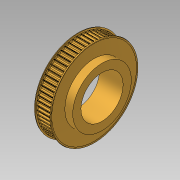
# Autodesk Inventor part: Engine Belt Wheel-2
Saved by Autodesk Inventor 2018.2 (Build 222227000, 227)
## iProperties
Created: 2019-08-01
Part Number: Engine Belt Wheel-2
Material: Generic
Document SubType Name: Modeling
Designer: NiveshandNisheeth
Density: 1 g/cm^3
Appearance: Brass - Satin
Author: NiveshandNisheeth
Autodesk Inventor part; units mm, degrees
ref_plane "YZ Plane" through (0, 0, 0) normal (1, 0, 0) x (0, 1, 0)
ref_plane "XZ Plane" through (0, 0, 0) normal (0, 1, 0) x (-1, 0, 0)
ref_plane "XY Plane" through (0, 0, 0) normal (0, 0, 1) x (1, 0, 0)
sketch "Sketch1" plane through (0, 0, 0) normal (1, 0, 0) x (0, 1, 0)
  line L0 (40, 0) -> (40, -45)
  line L1 (40, -45) -> (55.5, -45)
  line L2 (55.5, -45) -> (55.5, -30)
  line L3 (55.5, -30) -> (80, -30)
  line L4 (80, -30) -> (80, 0)
  line L5 (80, 0) -> (40, 0)
  line L6 (0, -54) -> (0, 9) projected
  point P0 (0, 0)
  dimension "d0" = 40
  dimension "d1" = 15.5
  dimension "d2" = 15
  dimension "d3" = 30
  dimension "d4" = 40
  constraints: 12 end point, 5 perpendicular, 1 horizontal alignment, 1 vertical
  measures "d0" distance from line of point (0, 0) L0
  measures "d1" distance of L0.end L1.end
  measures "d2" distance of L1.end L2.end
  measures "d3" distance of L3.end L4.end
  measures "d4" distance of L4.end L0.start
revolve "Revolution1" add sketch "Sketch1" angle 360 about axis through (0, 0, -10) along (0, 0, 1)
sketch "Sketch2" plane through (0, 0, 0) normal (0, 0, 1) x (1, 0, 0)
  arc A0 (-3, 79) -> (3, 79) centre (0, 79) ccw construction
  line L0 (-3.75, 81) -> (3.75, 81)
  line L1 (3.75, 81) -> (3.75, 79)
  line L2 (3.75, 79) -> (-3.75, 79) construction
  line L3 (-3.75, 79) -> (-3.75, 81)
  line L4 (-1.199, 76.25) -> (1.199, 76.25)
  line L5 (-3.75, 79) -> (-3.6742, 79)
  line L6 (3.6742, 79) -> (3.75, 79)
  arc A1 (-2.9394, 78.4) -> (-1.199, 76.25) centre (0, 79) ccw
  arc A2 (1.199, 76.25) -> (2.9394, 78.4) centre (0, 79) ccw
  arc A3 (-2.9394, 78.4) -> (-3.6742, 79) centre (-3.6742, 78.25) ccw
  arc A4 (3.6742, 79) -> (2.9394, 78.4) centre (3.6742, 78.25) ccw
  point P0 (0, 0)
  dimension "d6" = 3
  dimension "d7" = 2
  dimension "d8" = 7.5
  dimension "d9" = 79
  dimension "d10" = 2.75
  dimension "d11" = 0.75
  constraints: 14 end point, 14 point on circle, 5 centre point, 4 point on line, 4 tangent, 3 coincident, 3 equal length, 3 horizontal, 1 equal radius, 1 midpoint, 1 perpendicular, 1 vertical alignment
  measures "d6" radius of A0
  measures "d7" distance of L0.end L1.end
  measures "d8" distance of L0.start L0.end
  measures "d9" distance of point (0, 0) A0.centre
  measures "d10" distance from line of L4 A0.centre
  measures "d11" radius of A3
extrude "Extrusion1" cut sketch "Sketch2" against normal through all
pattern_circular "Circular Pattern1" count 64 over 360 about axis through (0, 0, -10) along (0, 0, 1) of "Extrusion1"
sketch "Sketch3" plane through (0, 0, 0) normal (1, 0, 0) x (0, 1, 0)
  line L0 (37.0014, 0) -> (-40, 0) construction
  line L1 (-40, 0) -> (-40, -45) construction
  line L2 (-40, -45) -> (-55.5, -45) construction
  line L3 (-55.5, -45) -> (-55.5, -30) construction
  line L4 (-55.5, -30) -> (37.0014, -30) construction
  line L5 (40, 0) -> (76.25, 0) construction
  line L6 (76.25, -30) -> (55.5, -30) construction
  line L7 (55.5, -30) -> (55.5, -45) construction
  line L8 (55.5, -45) -> (40, -45) construction
  line L9 (40, -45) -> (40, 0) construction
  line L10 (79.9121, 0) -> (79.9121, -30) construction
  line L11 (75.6121, 0) -> (80.6121, 0) construction
  line L12 (80.6121, 0) -> (80.6121, -1.5) construction
  line L13 (80.6121, -1.5) -> (75.6121, -1.5)
  line L14 (75.6121, -1.5) -> (75.6121, 0)
  line L15 (80.6121, -1.5) -> (80.2238, -0.0511) construction
  line L16 (80.2238, -0.0511) -> (82.6238, 0.592) construction
  line L17 (82.6238, 0.592) -> (83.0121, -0.8569)
  line L18 (83.0121, -0.8569) -> (80.6121, -1.5)
  line L19 (82.6238, 0.592) -> (80.4146, 0)
  line L20 (80.4146, 0) -> (75.6121, 0)
  line L21 (84.5014, -15) -> (37.0014, -15)
  line L22 (37.0014, 0) -> (37.0014, -30) construction
  line L23 (80.6121, -28.5) -> (75.6121, -28.5)
  line L24 (75.6121, -28.5) -> (75.6121, -30)
  line L25 (82.6238, -30.592) -> (83.0121, -29.1431)
  line L26 (83.0121, -29.1431) -> (80.6121, -28.5)
  line L27 (82.6238, -30.592) -> (80.4146, -30)
  line L28 (80.4146, -30) -> (75.6121, -30)
  line L29 (0, -48.1184) -> (0, 8.7104) projected
  line L30 (76.25, 0) -> (76.25, -30) projected
  line L31 (-76.25, -30) -> (-76.25, 0) projected
  point P0 (0, 0)
  dimension "d17" = 0.7
  dimension "d18" = 5
  dimension "d19" = 1.5
  dimension "d20" = 2.4
  dimension "d21" = 165
  dimension "d22" = 1.5
  constraints: 34 end point, 6 symmetric about line, 4 parallel, 3 perpendicular, 3 point on line, 2 horizontal, 1 midpoint, 1 other
  measures "d17" distance between parallel lines of L12 L10
  measures "d18" distance of L12.end L13.end
  measures "d19" distance of L13.end L11.start
  measures "d20" distance from line of L12 L17.end
  measures "d21" angle of L13 L18
  measures "d22" distance of L16.end L17.end
revolve "Revolution2" add sketch "Sketch3" angle 360 about axis through (0, 0, -10) along (0, 0, 1)
body "Solid1"
